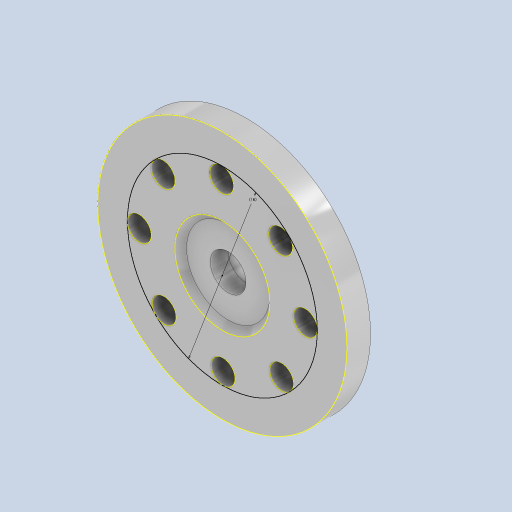
# Autodesk Inventor part: servohorn_zegi
Saved by Autodesk Inventor 2024 (Build 280153000, 153)
## iProperties
Created: 2023-08-25
Part Number: servohorn_zegi
Material: アルミニウム 6061-AHC
Document SubType Name: Modeling
Designer: zegi
Density: 2.7 g/cm^3
Appearance: アルミニウム - ダーク
Mass: 1.86596 g
Surface Area: 10.4255 cm^2
Volume: 0.691098 cm^3
Author: zegi
Autodesk Inventor part; units mm, degrees
ref_plane "YZ Plane" through (0, 0, 0) normal (1, 0, 0) x (0, 1, 0)
ref_plane "XZ Plane" through (0, 0, 0) normal (0, 1, 0) x (-1, 0, 0)
ref_plane "XY Plane" through (0, 0, 0) normal (0, 0, 1) x (1, 0, 0)
sketch "スケッチ1" plane through (0, 0, 0) normal (0, 0, 1) x (1, 0, 0)
  circle A0 centre (0, 0) radius 10.5
  circle A1 centre (0, 0) radius 3.5
  circle A2 centre (0, 0) radius 7 construction
  circle A3 centre (0, 0) radius 7 construction
  circle A4 centre (0, 0) radius 7 construction
  circle A5 centre (0, 0) radius 7 construction
  circle A6 centre (0, 0) radius 7 construction
  circle A7 centre (0, 0) radius 7 construction
  circle A8 centre (0, 0) radius 7 construction
  circle A9 centre (0, 0) radius 7 construction
  circle A10 centre (0, 0) radius 4
  circle A11 centre (0, 0) radius 1.5
  circle A12 centre (0, 0) radius 3
  point P0 (-0.061, 6.9997)
  point P1 (-4.9927, 4.9064)
  point P2 (-6.9997, -0.061)
  point P3 (-4.9064, -4.9927)
  point P4 (0.061, -6.9997)
  point P5 (4.9927, -4.9064)
  point P6 (6.9997, 0.061)
  point P7 (4.9064, 4.9927)
  dimension "d2" = 14
  dimension "d0" = 21
  dimension "d1" = 7
  dimension "d5" = 360
  dimension "d7" = 8
  dimension "d8" = 3
  dimension "d11" = 6
  constraints: 6 coincident, 5 centre point, 49 other
  measures "d0" diameter of A0
  measures "d1" diameter of A1
  measures "d7" diameter of A10
  measures "d8" diameter of A11
  measures "d11" diameter of A12
extrude "押し出し1" add sketch "スケッチ1" against normal blind 2 contours A0 | A1 | A10 | A12
extrude "押し出し2" add sketch "スケッチ1" against normal blind 5.7 contours A1 | A10
extrude "押し出し3" cut sketch "スケッチ1" against normal blind 0.5 contours A1 | A12
chamfer "面取り1" distance 0.5 angle 45 1 edges at (-3.5, 0, 0)
hole "穴1" at (-0.061, 6.9997, 0) at (-4.9927, 4.9064, 0) at (-6.9997, -0.061, 0) at (-4.9064, -4.9927, 0) at (0.061, -6.9997, 0) at (4.9927, -4.9064, 0) at (6.9997, 0.061, 0) at (4.9064, 4.9927, 0) direction (0, 0, -1) diameter 2 end through all
sketch "スケッチ2" plane through (0, 0, 0) normal (0, 0, 1) x (1, 0, 0)
  circle A0 centre (4.9064, 4.9927) radius 1 projected
  circle A1 centre (6.9997, 0.061) radius 1 projected
  circle A2 centre (4.9927, -4.9064) radius 1 projected
  circle A3 centre (0.061, -6.9997) radius 1 projected
  circle A4 centre (-4.9064, -4.9927) radius 1 projected
  circle A5 centre (-6.9997, -0.061) radius 1 projected
  circle A6 centre (-4.9927, 4.9064) radius 1 projected
  circle A7 centre (-0.061, 6.9997) radius 1 projected
  circle A8 centre (0, 0) radius 10.5 projected
  circle A9 centre (0, 0) radius 4 projected
  circle A10 centre (0, 0) radius 8
  circle A11 centre (-0.061, 6.9997) radius 1 projected
  dimension "d26" = 16
  constraints: 1 centre point, 1 coincident, 1 tangent
  measures "d26" diameter of A10
